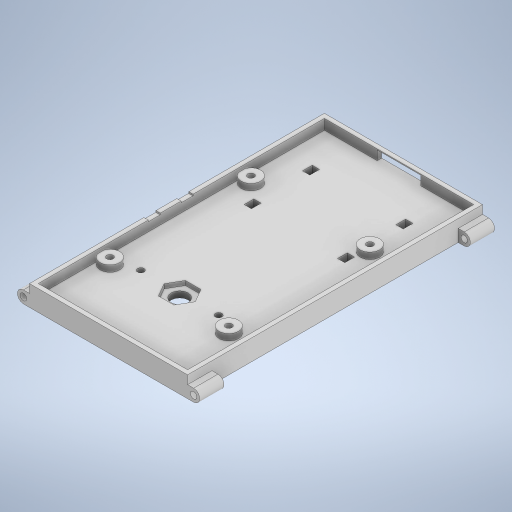
# Autodesk Inventor part: BOT
Saved by Autodesk Inventor 2023.1 (Build 271208000, 208)
## iProperties
Created: 2023-01-29
Part Number: BOT
Material: Generic
Document SubType Name: Modeling
Designer: liaar
Density: 1 g/cm^3
Appearance: Default
Author: liaar
Autodesk Inventor part; units mm, degrees
ref_plane "YZ Plane" through (0, 0, 0) normal (1, 0, 0) x (0, 1, 0)
ref_plane "XZ Plane" through (0, 0, 0) normal (0, 1, 0) x (-1, 0, 0)
ref_plane "XY Plane" through (0, 0, 0) normal (0, 0, 1) x (1, 0, 0)
sketch "Sketch2" plane through (0, 0, 0) normal (0, 1, 0) x (-1, 0, 0)
  line L0 (0, 0) -> (-65, 0)
  line L1 (-65, 0) -> (-65, -121.25)
  line L2 (-65, -121.25) -> (0, -121.25)
  line L3 (0, -121.25) -> (0, 0)
  line L4 (-1.8, -119.45) -> (-63.2, -119.45)
  line L5 (-63.2, -119.45) -> (-63.2, -1.8)
  line L6 (-63.2, -1.8) -> (-1.8, -1.8)
  line L7 (-1.8, -1.8) -> (-1.8, -119.45)
  dimension "d0" = 121.25
  dimension "d1" = 65
  dimension "d2" = 1.8
  dimension "d3" = 1.8
  dimension "d4" = 1.8
  dimension "d5" = 1.8
  constraints: 16 end point, 4 parallel, 2 horizontal, 2 perpendicular
  measures "d0" distance of L2.end L0.start
  measures "d1" distance of L1.end L2.end
  measures "d2" distance between parallel lines of L3 L7
  measures "d3" distance between parallel lines of L1 L5
  measures "d4" distance between parallel lines of L2 L4
  measures "d5" distance between parallel lines of L0 L6
extrude "Extrusion1" add sketch "Sketch2" along normal blind 6
extrude "Extrusion2" add sketch "Sketch2" along normal blind 1.8 contours L4 L5 L6 L7
sketch "Sketch3" plane through (0, 1.8, 0) normal (0, 1, 0) x (1, 0, 0)
  circle A0 centre (5.5, 27.55) radius 1.35
  circle A1 centre (54.4, 27.55) radius 1.35
  circle A2 centre (5.5, 85.55) radius 1.35
  circle A3 centre (54.4, 85.55) radius 1.35
  line L0 (63.2, 1.8) -> (1.8, 1.8) projected
  line L1 (1.8, 1.8) -> (1.8, 119.45) projected
  line L2 (1.8, 1.8) -> (1.8, 119.45) projected
  line L3 (63.2, 119.45) -> (63.2, 1.8) projected
  line L4 (1.8, 119.45) -> (63.2, 119.45) projected
  line L5 (1.8, 119.45) -> (9.8, 119.45)
  line L6 (1.8, 111.45) -> (1.8, 119.45)
  line L7 (63.2, 111.45) -> (63.2, 119.45)
  point P0 (0, 0)
  point P1 (63.2, 31.55)
  dimension "d10" = 25.75
  dimension "d11" = 2.7
  dimension "d12" = 2.7
  dimension "d13" = 2.7
  dimension "d14" = 2.7
  dimension "d17" = 3.7
  dimension "d20" = 58
  dimension "d21" = 58
  dimension "d45" = 48.9
  constraints: 6 end point, 4 centre point, 2 vertical alignment, 1 horizontal, 1 horizontal alignment, 1 point on line
  measures "d10" distance from line of L0 A0.centre
  measures "d11" diameter of A0
  measures "d12" diameter of A1
  measures "d13" diameter of A2
  measures "d14" diameter of A3
  measures "d17" distance from line of L1 A0.centre
  measures "d20" distance of A2.centre A0.centre
  measures "d21" distance of A1.centre A3.centre
  measures "d45" distance of A1.centre A0.centre
extrude "Extrusion4" cut sketch "Sketch3" against normal through all contours A0 | A1 | A2 | A3
sketch "Sketch4" plane through (0, 6, 0) normal (0, 1, 0) x (1, 0, 0)
  line L0 (0, 121.25) -> (0, 0) projected
  line L1 (1.8, 1.8) -> (1.8, 119.45) projected
  line L2 (0, 65.45) -> (1.8, 65.45)
  line L3 (1.8, 65.45) -> (1.8, 60.55)
  line L4 (1.8, 60.55) -> (0, 60.55)
  line L5 (0, 60.55) -> (0, 65.45)
  line L6 (0, 51.95) -> (1.8, 51.95)
  line L7 (1.8, 51.95) -> (1.8, 47.05)
  line L8 (1.8, 47.05) -> (0, 47.05)
  line L9 (0, 47.05) -> (0, 51.95)
  line L10 (65, 121.25) -> (0, 121.25) projected
  line L11 (0, 0) -> (65, 0) projected
  point P0 (1.8, 31.55)
  point P1 (1.8, 81.45)
  point P2 (1.8, 29.0699)
  dimension "d33" = 4.9
  dimension "d34" = 8.6
  dimension "d35" = 4.9
  dimension "d52" = 47.05
  constraints: 16 end point, 4 parallel, 4 point on line, 2 horizontal, 2 perpendicular
  measures "d33" distance of L3.end L2.end
  measures "d34" distance between parallel lines of L6 L4
  measures "d35" distance of L7.end L6.end
  measures "d52" distance between parallel lines of L11 L8
extrude "Extrusion5" cut sketch "Sketch4" against normal blind 0.6 contours L2 L1 L4 L0 | L6 L1 L8 L0
sketch "Sketch5" plane through (65, 0, -121.25) normal (0, 0, -1) x (-1, 0, 0)
  line L0 (23.5, 5.6) -> (41.5, 5.6)
  line L1 (41.5, 5.6) -> (41.5, 1.8)
  line L2 (41.5, 1.8) -> (23.5, 1.8)
  line L3 (23.5, 1.8) -> (23.5, 5.6)
  line L4 (65, 0) -> (65, 6) projected
  line L5 (0, 0) -> (0, 6) projected
  line L6 (0, 6) -> (65, 6) projected
  dimension "d38" = 23.5
  dimension "d39" = 23.5
  dimension "d40" = 0.4
  dimension "d41" = 3.8
  constraints: 8 end point, 2 parallel, 1 horizontal, 1 perpendicular
  measures "d38" distance between parallel lines of L4 L1
  measures "d39" distance between parallel lines of L5 L3
  measures "d40" distance between parallel lines of L6 L0
  measures "d41" distance of L2.end L0.start
extrude "Extrusion6" cut sketch "Sketch5" against normal up to surface (1.8 mm away)
sketch "Sketch6" plane through (0, 1.8, 0) normal (0, 1, 0) x (1, 0, 0)
  line L0 (33.1543, 26.25) -> (26.7457, 26.25)
  line L1 (26.7457, 26.25) -> (23.5414, 31.8)
  line L2 (23.5414, 31.8) -> (26.7457, 37.35)
  line L3 (26.7457, 37.35) -> (33.1543, 37.35)
  line L4 (33.1543, 37.35) -> (36.3586, 31.8)
  line L5 (36.3586, 31.8) -> (33.1543, 26.25)
  line L6 (63.2, 1.8) -> (1.8, 1.8) projected
  circle A0 centre (5.5, 27.55) radius 1.35 projected
  point P0 (0, 0)
  point P1 (29.95, 31.8)
  dimension "d46" = 11.1
  dimension "d47" = 30
  dimension "d48" = 24.45
  constraints: 12 end point, 1 horizontal, 13 other
  measures "d46" distance between parallel lines of L0 L3
  measures "d47" distance from line of L6 point (29.95, 31.8)
  measures "d48" horizontal distance of A0.centre point (29.95, 31.8)
extrude "Extrusion7" cut sketch "Sketch6" against normal blind 2.5 contours L0 L1 L2 L3 L4 L5
sketch "Sketch7" plane through (0, 1.8, 0) normal (0, 1, 0) x (1, 0, 0)
  line L0 (23.5414, 31.8) -> (26.7457, 26.25) projected
  line L1 (33.1543, 26.25) -> (26.7457, 26.25) projected
  line L2 (26.7457, 26.25) -> (33.1543, 26.25)
  line L3 (11.8, 104.45) -> (14.8, 104.45)
  line L4 (14.8, 104.45) -> (14.8, 100.45)
  line L5 (14.8, 100.45) -> (11.8, 100.45)
  line L6 (11.8, 100.45) -> (11.8, 104.45)
  line L7 (11.8, 80.45) -> (14.8, 80.45)
  line L8 (14.8, 80.45) -> (14.8, 76.45)
  line L9 (14.8, 76.45) -> (11.8, 76.45)
  line L10 (11.8, 76.45) -> (11.8, 80.45)
  line L11 (1.8, 119.45) -> (63.2, 119.45) projected
  line L12 (1.8, 65.45) -> (1.8, 119.45) projected
  line L13 (53.2, 104.45) -> (50.2, 104.45)
  line L14 (50.2, 104.45) -> (50.2, 100.45)
  line L15 (50.2, 100.45) -> (53.2, 100.45)
  line L16 (53.2, 100.45) -> (53.2, 104.45)
  line L17 (53.2, 80.45) -> (50.2, 80.45)
  line L18 (50.2, 80.45) -> (50.2, 76.45)
  line L19 (50.2, 76.45) -> (53.2, 76.45)
  line L20 (53.2, 76.45) -> (53.2, 80.45)
  circle A0 centre (5.5, 85.55) radius 1.35 projected
  line L21 (63.2, 119.45) -> (63.2, 1.8) projected
  point P0 (0, 0)
  point P1 (53.2, 102.45)
  point P2 (53.2, 78.45)
  point P3 (51.7, 104.45)
  point P4 (13.3, 104.45)
  point P5 (51.7, 80.45)
  point P6 (13.3, 80.45)
  point P7 (51.7, 76.45)
  point P8 (13.3, 76.45)
  point P9 (51.7, 100.45)
  point P10 (13.3, 100.45)
  dimension "d53" = 3
  dimension "d54" = 4
  dimension "d55" = 15
  dimension "d57" = 10
  dimension "d63" = 20
  dimension "d65" = 10
  dimension "d66" = 3
  dimension "d68" = 90
  constraints: 34 end point, 12 equal length, 10 midpoint, 4 horizontal alignment, 4 point on line, 2 horizontal, 2 perpendicular, 1 vertical alignment
  measures "d53" distance of L3.start L3.end
  measures "d54" distance of L5.end L3.start
  measures "d55" distance between parallel lines of L11 L3
  measures "d57" distance between parallel lines of L12 L6
  measures "d63" distance between parallel lines of L7 L5
  measures "d65" distance between parallel lines of L21 L16
  measures "d66" distance of L13.start L14.start
  measures "d68" angle of L16 L15
extrude "Extrusion8" cut sketch "Sketch7" against normal up to surface (1.8 mm away) contours L3 L4 L5 L6 | L7 L8 L9 L10 | L16 L15 L14 L13 | L20 L19 L18 L17
sketch "Sketch8" plane through (0, 0, 0) normal (0, -1, 0) x (1, 0, 0)
  line L0 (65, 0) -> (65, -121.25) projected
  line L1 (0, -121.25) -> (0, 0) projected
  line L2 (65, -121.25) -> (0, -121.25)
  line L3 (0, -121.25) -> (0, 0)
  line L4 (0, 0) -> (65, 0)
  line L5 (65, 0) -> (65, -121.25)
  line L6 (26.7457, -26.25) -> (33.1543, -26.25) projected
  line L7 (33.1543, -26.25) -> (36.3586, -31.8) projected
  line L8 (36.3586, -31.8) -> (33.1543, -37.35) projected
  line L9 (33.1543, -37.35) -> (26.7457, -37.35) projected
  line L10 (26.7457, -37.35) -> (23.5414, -31.8) projected
  line L11 (23.5414, -31.8) -> (26.7457, -26.25) projected
  circle A0 centre (29.95, -31.8) radius 5.55
  circle A1 centre (13.95, -31.8) radius 1.35
  circle A2 centre (45.95, -31.8) radius 1.35
  line L12 (53.2, -100.45) -> (53.2, -104.45) projected
  line L13 (53.2, -104.45) -> (50.2, -104.45) projected
  line L14 (50.2, -104.45) -> (50.2, -100.45) projected
  line L15 (50.2, -100.45) -> (53.2, -100.45) projected
  line L16 (11.8, -80.45) -> (11.8, -76.45) projected
  line L17 (11.8, -76.45) -> (14.8, -76.45) projected
  line L18 (14.8, -76.45) -> (14.8, -80.45) projected
  line L19 (14.8, -80.45) -> (11.8, -80.45) projected
  line L20 (11.8, -100.45) -> (14.8, -100.45) projected
  line L21 (14.8, -100.45) -> (14.8, -104.45) projected
  line L22 (14.8, -104.45) -> (11.8, -104.45) projected
  line L23 (11.8, -104.45) -> (11.8, -100.45) projected
  line L24 (50.2, -76.45) -> (53.2, -76.45) projected
  line L25 (53.2, -76.45) -> (53.2, -80.45) projected
  line L26 (53.2, -80.45) -> (50.2, -80.45) projected
  line L27 (50.2, -80.45) -> (50.2, -76.45) projected
  circle A3 centre (5.5, -85.55) radius 1.35 projected
  circle A4 centre (5.5, -27.55) radius 1.35 projected
  circle A5 centre (54.4, -85.55) radius 1.35 projected
  circle A6 centre (54.4, -27.55) radius 1.35 projected
  line L28 (65, 0) -> (65, -121.25) projected
  line L29 (0, 0) -> (65, 0) projected
  line L30 (0, -121.25) -> (0, 0) projected
  line L31 (65, -121.25) -> (0, -121.25) projected
  line L32 (53.2, -104.45) -> (53.2, -100.45) projected
  line L33 (50.2, -104.45) -> (50.2, -100.45) projected
  line L34 (53.2, -104.45) -> (50.2, -104.45)
  line L35 (50.2, -104.45) -> (50.2, -100.45)
  line L36 (50.2, -100.45) -> (53.2, -100.45)
  line L37 (53.2, -100.45) -> (53.2, -104.45)
  line L38 (50.2, -80.45) -> (53.2, -80.45) projected
  line L39 (50.2, -76.45) -> (50.2, -80.45) projected
  line L40 (53.2, -80.45) -> (50.2, -80.45)
  line L41 (50.2, -80.45) -> (50.2, -76.45)
  line L42 (50.2, -76.45) -> (53.2, -76.45)
  line L43 (53.2, -76.45) -> (53.2, -80.45)
  line L44 (11.8, -76.45) -> (14.8, -76.45) projected
  line L45 (14.8, -80.45) -> (11.8, -80.45)
  line L46 (11.8, -80.45) -> (11.8, -76.45)
  line L47 (11.8, -76.45) -> (14.8, -76.45)
  line L48 (14.8, -76.45) -> (14.8, -80.45)
  line L49 (14.8, -104.45) -> (11.8, -104.45)
  line L50 (11.8, -104.45) -> (11.8, -100.45)
  line L51 (11.8, -100.45) -> (14.8, -100.45)
  line L52 (14.8, -100.45) -> (14.8, -104.45)
  circle A7 centre (54.4, -85.55) radius 1.35 projected
  circle A8 centre (54.4, -85.55) radius 1.35
  circle A9 centre (5.5, -85.55) radius 1.35 projected
  circle A10 centre (5.5, -85.55) radius 1.35
  dimension "d69" = 11.1
  dimension "d70" = 16
  dimension "d71" = 13.95
  dimension "d72" = 35.05
  dimension "d73" = 31.8
  dimension "d74" = 16
  dimension "d75" = 2.7
  dimension "d76" = 2.7
  dimension "d77" = 19.05
  dimension "d78" = 2.7
  dimension "d81" = 2.7
  constraints: 40 end point, 10 parallel, 5 centre point, 5 horizontal, 5 perpendicular, 2 coincident
  measures "d69" diameter of A0
  measures "d70" distance of A1.centre A0.centre
  measures "d71" distance from line of L1 A1.centre
  measures "d72" distance from line of L0 A0.centre
  measures "d73" distance from line of L4 A0.centre
  measures "d74" distance of A2.centre A0.centre
  measures "d75" diameter of A2
  measures "d76" diameter of A1
  measures "d77" distance from line of L0 A2.centre
  measures "d78" diameter of A10
  measures "d81" diameter of A8
extrude "Extrusion9" add sketch "Sketch8" along normal blind 2.5 contours L0 L2 L1 L4 | L6 A0 L11 | L6 L7 A0 | A0 | A0 L10 L11 | L7 L8 A0 | A0 L9 L10 | A0 L8 L9
extrude "Extrusion10" cut sketch "Sketch8" against normal blind 2 contours A1 | A2
sketch "Sketch9" plane through (0, 1.8, 0) normal (0, 1, 0) x (1, 0, 0)
  circle A0 centre (29.95, 31.8) radius 3.5
  line L0 (23.5414, 31.8) -> (26.7457, 26.25) projected
  line L1 (25.1436, 29.025) -> (34.7564, 34.575) construction
  line L2 (33.1543, 37.35) -> (36.3586, 31.8) projected
  point P0 (0, 0)
  dimension "d84" = 7
  constraints: 3 midpoint, 2 end point, 1 centre point, 1 coincident
  measures "d84" diameter of A0
extrude "Extrusion11" cut sketch "Sketch9" against normal up to surface (4.3 mm away)
sketch "Sketch10" plane through (0, 1.8, 0) normal (0, 1, 0) x (1, 0, 0)
  circle A0 centre (54.4, 85.55) radius 1.35 projected
  circle A1 centre (54.4, 85.55) radius 4
  circle A2 centre (5.5, 85.55) radius 1.35 projected
  circle A3 centre (5.5, 85.55) radius 4
  circle A4 centre (54.4, 27.55) radius 1.35 projected
  circle A5 centre (54.4, 27.55) radius 4
  circle A6 centre (5.5, 27.55) radius 1.35 projected
  circle A7 centre (5.5, 27.55) radius 4
  circle A8 centre (54.4, 85.55) radius 1.35
  circle A9 centre (5.5, 85.55) radius 1.35
  circle A10 centre (5.5, 27.55) radius 1.35
  circle A11 centre (54.4, 27.55) radius 1.35
  point P0 (0, 0)
  dimension "d87" = 8
  dimension "d88" = 8
  dimension "d89" = 8
  dimension "d90" = 8
  constraints: 8 centre point, 8 coincident, 4 concentric
  measures "d87" diameter of A1
  measures "d88" diameter of A3
  measures "d89" diameter of A5
  measures "d90" diameter of A7
extrude "Extrusion12" add sketch "Sketch10" along normal blind 2.6
sketch "Sketch11" plane through (65, 6, -121.25) normal (0, 0, -1) x (-1, 0, 0)
  line L0 (65, -8.5) -> (0, -8.5) projected
  line L1 (65, -8.5) -> (70, -8.5)
  line L2 (70, -8.5) -> (70, -3.5)
  line L3 (70, -3.5) -> (65, -3.5)
  line L4 (65, -3.5) -> (65, -8.5)
  line L5 (0, -8.5) -> (0, 0) projected
  line L6 (0, -8.5) -> (-5, -8.5)
  line L7 (-5, -8.5) -> (-5, -3.5)
  line L8 (-5, -3.5) -> (0, -3.5)
  line L9 (0, -3.5) -> (0, -8.5)
  circle A0 centre (-2.5, -6) radius 1.35
  circle A1 centre (67.5, -6) radius 1.35
  point P0 (65, -6)
  point P1 (0, -6)
  point P2 (0, -3.5)
  dimension "d93" = 5
  dimension "d94" = 5
  dimension "d95" = 5
  dimension "d96" = 5
  dimension "d97" = 2.7
  dimension "d98" = 2.7
  dimension "d99" = 2.5
  dimension "d100" = 2.5
  dimension "d101" = 2.5
  dimension "d102" = 2.5
  dimension "d103" = 2.5
  constraints: 16 end point, 4 parallel, 2 centre point, 2 horizontal, 2 perpendicular, 1 midpoint
  measures "d93" distance of L0.start L1.end
  measures "d94" distance of L1.end L2.end
  measures "d95" distance of L0.end L6.end
  measures "d96" distance of L6.end L7.end
  measures "d97" diameter of A1
  measures "d98" diameter of A0
  measures "d99" distance of point (0, -6) A0.centre
  measures "d100" distance from line of L8 A0.centre
  measures "d101" distance from line of L4 A1.centre
  measures "d102" distance from line of L2 A1.centre
  measures "d103" distance from line of L1 A1.centre
extrude "Extrusion13" add sketch "Sketch11" against normal blind 10
sketch "Sketch12" plane through (0, 6, 0) normal (0, 0, 1) x (1, 0, 0)
  line L0 (-5, -3.5) -> (-5, -8.5) projected
  line L1 (-5, -8.5) -> (0, -8.5) projected
  line L2 (0, -3.5) -> (0, -8.5) projected
  line L3 (0, -3.5) -> (-5, -3.5) projected
  circle A0 centre (-2.5, -6) radius 1.35 projected
  line L4 (65, -8.5) -> (70, -8.5) projected
  line L5 (70, -8.5) -> (70, -3.5) projected
  line L6 (70, -3.5) -> (65, -3.5) projected
  line L7 (65, -8.5) -> (65, -3.5) projected
  circle A1 centre (67.5, -6) radius 1.35 projected
  point P0 (0, -6)
extrude "Extrusion14" add sketch "Sketch12" against normal blind 10
full round fillet "Full Round Fillet1" first side at (68.3333, 2.5, -3.3333) centre faces at (70, -0.8333, -3.3333) second side at (31.7906, -2.5, -62.7248)
full round fillet "Full Round Fillet2" first side at (-1.6667, 2.5, -3.3333) centre faces at (-5, 0.8333, -6.6667) second side at (32.624, -2.5, -12.7752)
full round fillet "Full Round Fillet3" first side at (-3.3333, 2.5, -117.9167) centre faces at (-5, -0.8333, -117.9167) second side at (31.7906, -2.5, -9.4418)
full round fillet "Full Round Fillet4" first side at (66.6667, 2.5, -117.9167) centre faces at (70, 0.8333, -117.9167) second side at (31.7906, -2.5, -9.4418)
body "Solid1"
